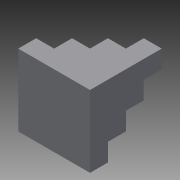
# Autodesk Inventor part: 157
Saved by Autodesk Inventor 2014 (Build 180170000, 170)
## iProperties
Created: 2017-04-22
Part Number: 157
Material: Generic
Document SubType Name: Modeling
Designer: Andy
Density: 1 g/cm^3
Appearance: Default
Author: Andy
Autodesk Inventor part; units mm, degrees
ref_plane "YZ Plane" through (0, 0, 0) normal (1, 0, 0) x (0, 1, 0)
ref_plane "XZ Plane" through (0, 0, 0) normal (0, 1, 0) x (-1, 0, 0)
ref_plane "XY Plane" through (0, 0, 0) normal (0, 0, 1) x (1, 0, 0)
sketch "Sketch1" plane through (0, 0, 0) normal (0, 1, 0) x (-1, 0, 0)
  line L0 (-5, 5) -> (5, 5)
  line L1 (5, 5) -> (5, -5)
  line L2 (5, -5) -> (-5, -5)
  line L3 (-5, -5) -> (-5, 5)
  line L4 (-5, 5) -> (5, -5) construction
  line L5 (5, 5) -> (-5, -5) construction
  point P0 (0, 0)
  dimension "d0" = 10
  dimension "d1" = 10
  constraints: 12 end point, 2 midpoint, 2 parallel, 1 horizontal, 1 perpendicular
  measures "d0" distance of L1.end L2.end
  measures "d1" distance of L0.end L1.end
extrude "Extrusion1" add sketch "Sketch1" along normal blind 10
sketch "Sketch2" plane through (5, 0, 5) normal (1, 0, 0) x (0, 0, -1)
  line L0 (10, 10) -> (7.5, 10)
  line L1 (7.5, 10) -> (7.5, 2.5)
  line L2 (7.5, 2.5) -> (10, 2.5)
  line L3 (10, 2.5) -> (10, 10)
  point P0 (5, 0)
  dimension "d4" = 2.5
  dimension "d5" = 7.5
  constraints: 8 end point, 2 parallel, 1 horizontal, 1 perpendicular
  measures "d4" distance of L2.end L1.end
  measures "d5" distance of L1.end L0.end
extrude "Extrusion2" cut sketch "Sketch2" against normal blind 10
sketch "Sketch3" plane through (5, 0, 5) normal (1, 0, 0) x (0, 0, -1)
  line L0 (7.5, 10) -> (5, 10)
  line L1 (5, 10) -> (5, 5)
  line L2 (5, 5) -> (7.5, 5)
  line L3 (7.5, 5) -> (7.5, 10)
  point P0 (5, 0)
  dimension "d8" = 2.5
  dimension "d9" = 5
  constraints: 8 end point, 2 parallel, 1 horizontal, 1 perpendicular
  measures "d8" distance of L2.end L1.end
  measures "d9" distance of L1.end L0.end
extrude "Extrusion3" cut sketch "Sketch3" against normal blind 10
sketch "Sketch4" plane through (5, 0, 5) normal (1, 0, 0) x (0, 0, -1)
  line L0 (5, 10) -> (2.5, 10)
  line L1 (2.5, 10) -> (2.5, 7.5)
  line L2 (2.5, 7.5) -> (5, 7.5)
  line L3 (5, 7.5) -> (5, 10)
  point P0 (5, 0)
  dimension "d12" = 2.5
  dimension "d13" = 2.5
  constraints: 8 end point, 2 parallel, 1 horizontal, 1 perpendicular
  measures "d12" distance of L2.end L1.end
  measures "d13" distance of L1.end L0.end
extrude "Extrusion4" cut sketch "Sketch4" against normal blind 10
sketch "Sketch5" plane through (-5, 0, 5) normal (0, 0, 1) x (1, 0, 0)
  line L0 (0, 10) -> (10, 10) projected
  line L1 (0, 0) -> (0, 10) projected
  line L2 (0, 10) -> (0, 2.5)
  line L3 (0, 2.5) -> (2.5, 2.5)
  line L4 (2.5, 2.5) -> (2.5, 5)
  line L5 (2.5, 5) -> (5, 5)
  line L6 (5, 5) -> (5, 7.5)
  line L7 (5, 7.5) -> (7.5, 7.5)
  line L8 (7.5, 7.5) -> (7.5, 10)
  point P0 (5, 0)
  dimension "d16" = 7.5
  dimension "d17" = 2.5
  dimension "d18" = 2.5
  dimension "d19" = 90
  dimension "d20" = 2.5
  dimension "d21" = 90
  dimension "d22" = 2.5
  dimension "d23" = 90
  dimension "d24" = 2.5
  dimension "d25" = 90
  constraints: 14 end point, 3 parallel, 3 perpendicular, 2 point on line
  measures "d16" distance of L0.start L2.end
  measures "d17" distance of L2.end L3.end
  measures "d18" distance of L3.end L4.end
  measures "d19" angle of L4 L3
  measures "d20" distance of L4.end L5.end
  measures "d21" angle of L4 L5
  measures "d22" distance of L5.end L6.end
  measures "d23" angle of L6 L5
  measures "d24" distance of L6.end L7.end
  measures "d25" angle of L6 L7
extrude "Extrusion5" cut sketch "Sketch5" against normal blind 10
body "Solid1"
